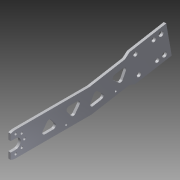
# Autodesk Inventor part: Arm_Link_1
Saved by Autodesk Inventor 2013 (Build 170138000, 138)
## iProperties
Created: 2014-05-15
Part Number: Arm_Link_1
Material: アルミニウム 6061
Document SubType Name: Modeling
Designer: andou
Density: 2.71 g/cm^3
Mass: 16.3631 g
Surface Area: 75.7922 cm^2
Volume: 6.03804 cm^3
Author: andou
Autodesk Inventor part; units mm, degrees
ref_plane "YZ Plane" through (0, 0, 0) normal (1, 0, 0) x (0, 1, 0)
ref_plane "XZ Plane" through (0, 0, 0) normal (0, 1, 0) x (-1, 0, 0)
ref_plane "XY Plane" through (0, 0, 0) normal (0, 0, 1) x (1, 0, 0)
sketch "スケッチ2" plane through (0, 0, 0) normal (1, 0, 0) x (0, 1, 0)
  line L0 (0, 0) -> (-59.3543, 0)
  line L1 (-59.3543, -20) -> (1.7498, -20)
  line L2 (0, 0) -> (58.4526, 10.3068)
  line L3 (61.9255, -9.3894) -> (1.7498, -20)
  arc A0 (62.5368, 10.1792) -> (58.4526, 10.3068) centre (60.1891, 0.4587) ccw
  arc A1 (61.9255, -9.3894) -> (65.7198, -7.8726) centre (60.1891, 0.4587) ccw
  arc A2 (-63.3543, -19.1652) -> (-59.3543, -20) centre (-59.3543, -10) ccw
  arc A3 (-59.3543, 0) -> (-63.3543, -0.8348) centre (-59.3543, -10) ccw
  arc A4 (-59.3543, -14) -> (-59.3543, -6) centre (-59.3543, -10) ccw
  line L4 (-59.3543, -6) -> (-63.3543, -6)
  line L5 (-59.3543, -14) -> (-63.3543, -14)
  line L6 (-63.3543, -0.8348) -> (-63.3543, -6)
  line L7 (-63.3543, -14) -> (-63.3543, -19.1652)
  line L8 (65.7198, -7.8726) -> (65.3114, -5.5567)
  line L9 (62.9451, 7.8632) -> (62.5368, 10.1792)
  line L10 (1.7498, -20) -> (0, 0)
  line L11 (65.3114, -5.5567) -> (62.9451, 7.8632)
  dimension "d21" = 20
  dimension "d22" = 10
  dimension "d23" = 170
  dimension "d27" = 10
  dimension "d31" = 8
  dimension "d33" = 4
  dimension "d35" = 4
  dimension "d36" = 120
  dimension "d139" = 20
  constraints: 24 end point, 10 point on circle, 8 perpendicular, 5 centre point, 4 equal length, 3 equal radius, 2 parallel, 2 tangent, 1 coincident, 1 collinear, 1 horizontal
  measures "d21" distance between parallel lines of L0 L1
  measures "d22" distance from line of L0 A2.centre
  measures "d23" angle of L0 L2
  measures "d27" radius of A3
  measures "d31" diameter of A4
  measures "d33" distance from line of L6 A2.centre
  measures "d35" distance from line of L8 L2.end
  measures "d36" distance of A2.centre A0.centre
  measures "d139" distance between parallel lines of L2 L3
extrude "押し出し1" add sketch "スケッチ2" along normal blind 2
sketch "スケッチ4" plane through (0, 0, 0) normal (-1, 0, 0) x (0, 0, 1)
  line L0 (-20, 1.7498) -> (-9.3894, 61.9255) projected
  line L1 (-20, -59.3543) -> (-20, 1.7498) projected
  circle A0 centre (-17, -18.5891) radius 1
  circle A1 centre (-13.5138, 21.2587) radius 1
  line L2 (-17, -18.5891) -> (-13.5138, 21.2587)
  line L3 (-20, 1.7498) -> (0, 0)
  dimension "d57" = 2
  dimension "d59" = 40
  dimension "d60" = 175
  dimension "d61" = 3
  dimension "d62" = 3
  constraints: 4 end point, 2 centre point, 1 equal radius
  measures "d57" diameter of A0
  measures "d59" distance of L2.start L2.end
  measures "d60" angle of L1 L2
  measures "d61" distance from line of L1 L2.start
  measures "d62" distance from line of L0 L2.end
hole "穴2" at (0, -18.5891, -17) at (0, 21.2587, -13.5138) direction (1, 0, 0) diameter 1.6 end through all
sketch "スケッチ6" plane through (2, 0, 0) normal (1, 0, 0) x (0, 0, -1)
  line L0 (20, 1.7498) -> (9.3894, 61.9255) projected
  arc A0 (9.3894, 61.9255) -> (7.8726, 65.7198) centre (-0.4587, 60.1891) ccw projected
  line L1 (7.8726, 65.7198) -> (-10.1792, 62.5368) projected
  arc A1 (-10.1792, 62.5368) -> (-10.3068, 58.4526) centre (-0.4587, 60.1891) ccw projected
  line L2 (-10.3068, 58.4526) -> (0, 0) projected
  line L3 (-5.04, 28.5832) -> (-8.2539, 32.4135)
  line L4 (-10.1792, 62.5368) -> (-13.4634, 61.9577)
  line L5 (-13.4634, 61.9577) -> (-8.2539, 32.4135)
  line L6 (7.8726, 65.7198) -> (11.1568, 66.2989)
  line L7 (11.1568, 66.2989) -> (16.3663, 36.7547)
  line L8 (16.3663, 36.7547) -> (14.6562, 32.0562)
  dimension "d75" = 150
  dimension "d76" = 150
  dimension "d77" = 2.5
  dimension "d78" = 2.5
  dimension "d79" = 30
  constraints: 12 end point, 3 parallel, 2 collinear, 2 point on line
  measures "d75" angle of L2 L3
  measures "d76" angle of L0 L8
  measures "d77" distance between parallel lines of L0 L7
  measures "d78" distance between parallel lines of L2 L5
  measures "d79" distance of L4.end L3.end
extrude "押し出し2" add sketch "スケッチ6" against normal blind 2
sketch "スケッチ5" plane through (2, 0, 0) normal (1, 0, 0) x (0, 0, -1)
  line L0 (7.8726, 65.7198) -> (-10.1792, 62.5368) projected
  circle A0 centre (-8.1635, 57.8151) radius 1.5
  circle A1 centre (7.5934, 60.5934) radius 1.5
  line L1 (14.6562, 32.0562) -> (20, 1.7498) projected
  line L2 (20, 1.7498) -> (20, -59.3543) projected
  arc A2 (19.1652, -63.3543) -> (20, -59.3543) centre (10, -59.3543) ccw projected
  line L3 (19.1652, -63.3543) -> (14, -63.3543) projected
  line L4 (14, -63.3543) -> (14, -59.3543) projected
  arc A3 (14, -59.3543) -> (6, -59.3543) centre (10, -59.3543) ccw projected
  line L5 (6, -59.3543) -> (6, -63.3543) projected
  line L6 (6, -63.3543) -> (0.8348, -63.3543) projected
  arc A4 (0, -59.3543) -> (0.8348, -63.3543) centre (10, -59.3543) ccw projected
  line L7 (0, -59.3543) -> (0, 0) projected
  line L8 (0, 0) -> (-5.04, 28.5832) projected
  circle A5 centre (17, -18.5891) radius 0.8 projected
  circle A6 centre (13.5138, 21.2587) radius 0.8 projected
  line L9 (-8.2539, 32.4135) -> (-13.4634, 61.9577) projected
  line L10 (-13.4634, 61.9577) -> (11.1568, 66.2989) projected
  line L11 (11.1568, 66.2989) -> (16.3663, 36.7547) projected
  line L12 (16.3663, 36.7547) -> (14.6562, 32.0562) projected
  line L13 (-5.04, 28.5832) -> (-8.2539, 32.4135) projected
  point P0 (3.5148, 90.434)
  point P1 (-14.537, 87.251)
  point P2 (-10.1792, 62.5368)
  dimension "d72" = 3
  dimension "d114" = 16
  dimension "d174" = 5
  dimension "d175" = 5
  dimension "d176" = 4.5
  constraints: 2 centre point, 1 equal radius, 1 other
  measures "d72" diameter of A1
  measures "d114" distance of A1.centre A0.centre
  measures "d174" distance from line of L10 A0.centre
  measures "d176" distance from line of L11 A1.centre
hole "穴3" at (2, 57.8151, 8.1635) at (2, 60.5934, -7.5934) direction (-1, 0, 0) diameter 4 end through all
sketch "スケッチ7" plane through (2, 0, 0) normal (1, 0, 0) x (0, 0, -1)
  arc A0 (0, -59.3543) -> (0.8348, -63.3543) centre (10, -59.3543) ccw projected
  line L0 (0.8348, -63.3543) -> (6, -63.3543) projected
  circle A1 centre (3, -59.3543) radius 1
  dimension "d89" = 4
  dimension "d90" = 7
  dimension "d91" = 2
  constraints: 1 centre point
  measures "d89" distance from line of L0 A1.centre
  measures "d90" distance of A1.centre A0.centre
  measures "d91" diameter of A1
hole "穴4" at (2, -59.3543, -3) direction (-1, 0, 0) diameter 2 end through all
pattern_circular "円形状パターン3" count 5 over 180 about axis through (0, -59.3543, -10) along (-1, 0, 0) of "穴4"
sketch "スケッチ8" plane through (2, 0, 0) normal (1, 0, 0) x (0, 0, -1)
  line L0 (11.1568, 66.2989) -> (-13.4634, 61.9577) projected
  line L1 (-13.4634, 61.9577) -> (-8.2539, 32.4135) projected
  circle A0 centre (-7.1216, 51.9062) radius 1.5
  circle A1 centre (8.6353, 54.6846) radius 1.5
  point P0 (7.8726, 65.7198)
  point P1 (-10.1792, 62.5368)
  dimension "d102" = 11
  dimension "d103" = 11
  dimension "d104" = 16
  dimension "d105" = 4.5
  dimension "d106" = 3
  constraints: 2 centre point, 1 equal radius
  measures "d102" distance from line of L0 A0.centre
  measures "d103" distance from line of L0 A1.centre
  measures "d104" distance of A1.centre A0.centre
  measures "d105" distance from line of L1 A0.centre
  measures "d106" diameter of A1
hole "穴5" at (2, 51.9062, 7.1216) at (2, 54.6846, -8.6353) direction (-1, 0, 0) diameter 3.5 end through all
sketch "スケッチ11" plane through (2, 0, 0) normal (1, 0, 0) x (0, 0, -1)
  circle A0 centre (-7.1216, 51.9062) radius 1.75 projected
  circle A1 centre (8.6353, 54.6846) radius 1.75 projected
  line L0 (-13.4634, 61.9577) -> (-8.2539, 32.4135) projected
  circle A2 centre (-4.5169, 37.1341) radius 1.5
  circle A3 centre (11.24, 39.9125) radius 1.5
  dimension "d124" = 3
  dimension "d126" = 16
  dimension "d127" = 15
  dimension "d128" = 4.5
  dimension "d130" = 15
  constraints: 2 centre point, 1 equal radius
  measures "d124" diameter of A2
  measures "d126" distance of A3.centre A2.centre
  measures "d127" distance of A0.centre A2.centre
  measures "d128" distance from line of L0 A2.centre
  measures "d130" distance of A1.centre A3.centre
hole "穴6" at (2, 37.1341, 4.5169) at (2, 39.9125, -11.24) direction (-1, 0, 0) diameter 3.5 end through all
sketch "スケッチ13" plane through (2, 0, 0) normal (1, 0, 0) x (0, 0, -1)
  line L0 (0, 0) -> (0, -59.3543) projected
  line L1 (20, -59.3543) -> (20, 1.7498) projected
  line L2 (20, 1.7498) -> (14.6562, 32.0562) projected
  line L3 (11.1568, 66.2989) -> (-13.4634, 61.9577) projected
  line L4 (-5.04, 28.5832) -> (0, 0) projected
  line L5 (-0.4338, 31.2538) -> (10.7167, 25.6042)
  line L6 (10.7167, 25.6042) -> (2.171, 16.4817)
  line L7 (2.171, 16.4817) -> (-0.4338, 31.2538)
  line L8 (4.2547, 4.664) -> (12.8005, 13.7865)
  line L9 (12.8005, 13.7865) -> (15.4052, -0.9856)
  line L10 (15.4052, -0.9856) -> (4.2547, 4.664)
  line L11 (5, -5.4856) -> (15, -12.9856)
  line L12 (5, -20.4856) -> (5, -5.4856)
  line L13 (15, -12.9856) -> (5, -20.4856)
  line L14 (5, -32.4856) -> (15, -24.9856)
  line L15 (15, -24.9856) -> (15, -39.9856)
  line L16 (15, -39.9856) -> (5, -32.4856)
  point P0 (9.3894, 61.9255)
  point P1 (7.8726, 65.7198)
  point P2 (-10.1792, 62.5368)
  point P3 (-10.3068, 58.4526)
  dimension "d147" = 5
  dimension "d149" = 5
  dimension "d160" = 5
  dimension "d162" = 40
  dimension "d163" = 52
  dimension "d164" = 12
  dimension "d166" = 5
  dimension "d177" = 10
  dimension "d178" = 15
  dimension "d179" = 12
  constraints: 24 end point, 10 equal length, 4 parallel
  measures "d147" distance between parallel lines of L4 L7
  measures "d149" distance between parallel lines of L9 L2
  measures "d160" distance between parallel lines of L12 L0
  measures "d162" distance from line of L3 L5.end
  measures "d163" distance from line of L3 L8.end
  measures "d164" vertical distance of L9.end L11.end
  measures "d166" distance between parallel lines of L1 L15
  measures "d177" distance from line of L7 L5.end
  measures "d178" distance of L6.end L5.start
  measures "d179" distance of L11.end L14.end
extrude "押し出し5" cut sketch "スケッチ13" against normal blind 2
fillet "フィレット2" radius 2 12 edges at (1, -24.9856, -15) (1, 13.7865, -12.8005) (1, 31.2538, 0.4338) (1, -5.4856, -5) (1, 4.664, -4.2547) (1, -32.4856, -5) (1, 25.6042, -10.7167) (1, -12.9856, -15) (1, -0.9856, -15.4052) (1, -39.9856, -15) (1, -20.4856, -5) (1, 16.4817, -2.171)
